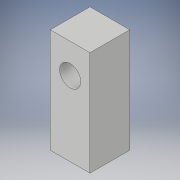
# Autodesk Inventor part: clevis
Saved by Autodesk Inventor 2017 (Build 210142000, 142)
## iProperties
Created: 2016-11-16
Part Number: clevis
Material: Generic
Document SubType Name: Modeling
Designer: gus
Density: 1 g/cm^3
Appearance: Default
Author: gus
Autodesk Inventor part; units mm, degrees
ref_plane "YZ Plane" through (0, 0, 0) normal (1, 0, 0) x (0, 1, 0)
ref_plane "XZ Plane" through (0, 0, 0) normal (0, 1, 0) x (-1, 0, 0)
ref_plane "XY Plane" through (0, 0, 0) normal (0, 0, 1) x (1, 0, 0)
sketch "Sketch1" plane through (0, 0, 0) normal (0, 1, 0) x (-1, 0, 0)
  circle A0 centre (0, 0) radius 3.175
  line L0 (6.35, 6.35) -> (-6.35, 6.35)
  line L1 (-6.35, 6.35) -> (-6.35, -6.35)
  line L2 (-6.35, -6.35) -> (6.35, -6.35)
  line L3 (6.35, -6.35) -> (6.35, 6.35)
  dimension "d0" = 6.35
  dimension "d1" = 6.35
  dimension "d2" = 6.35
  dimension "d3" = 6.35
  constraints: 8 end point, 2 parallel, 2 perpendicular, 1 centre point, 1 coincident, 1 horizontal
  measures "d0" diameter of A0
  measures "d1" distance from line of point (0, 0) L2
  measures "d2" distance from line of point (0, 0) L0
  measures "d3" distance from line of L1 point (0, 0)
extrude "Extrusion1" add sketch "Sketch1" along normal blind 30.1752 contours A0 | L3 L2 L1 L0
extrude "Extrusion2" cut sketch "Sketch1" along normal blind 12.7 contours A0
sketch "Sketch2" plane through (-6.35, 0, 6.35) normal (0, 0, 1) x (1, 0, 0)
  circle A0 centre (6.35, 23.8125) radius 3.3782
  line L0 (12.7, 0) -> (12.7, 30.1752) projected
  point P0 (6.35, 0)
  dimension "d8" = 6.7564
  dimension "d9" = 23.8125
  dimension "d10" = 6.35
  constraints: 1 centre point
  measures "d8" diameter of A0
  measures "d9" distance of A0.centre point (6.35, 0)
  measures "d10" distance from line of L0 A0.centre
extrude "Extrusion3" cut sketch "Sketch2" against normal blind 12.7
sketch "Sketch3" plane through (0, 30.1752, 0) normal (0, 1, 0) x (1, 0, 0)
  line L0 (6.35, -6.35) -> (6.35, 6.35) projected
  line L1 (6.35, 6.35) -> (-6.35, 6.35) projected
  line L2 (-6.35, 6.35) -> (-6.35, -6.35) projected
  line L3 (-6.35, -6.35) -> (6.35, -6.35) projected
  point P0 (0, 0)
extrude "Extrusion4" add sketch "Sketch3" along normal blind 3.175
body "Solid1"
